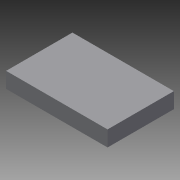
# Autodesk Inventor part: arduinoshape
Saved by Autodesk Inventor 2015 (Build 190159000, 159)
## iProperties
Created: 2015-01-29
Part Number: arduinoshape
Material: Generic
Document SubType Name: Modeling
Designer: robotics
Density: 1 g/cm^3
Appearance: Default
Author: robotics
Autodesk Inventor part; units mm, degrees
ref_plane "YZ Plane" through (0, 0, 0) normal (1, 0, 0) x (0, 1, 0)
ref_plane "XZ Plane" through (0, 0, 0) normal (0, 1, 0) x (-1, 0, 0)
ref_plane "XY Plane" through (0, 0, 0) normal (0, 0, 1) x (1, 0, 0)
sketch "Sketch2" plane through (0, 0, 0) normal (0, 1, 0) x (-1, 0, 0)
  line L0 (0, 0) -> (82.55, 0)
  line L1 (82.55, 0) -> (82.55, -53.975)
  line L2 (82.55, -53.975) -> (0, -53.975)
  line L3 (0, -53.975) -> (0, 0)
  dimension "d3" = 82.55
  dimension "d4" = 53.975
  constraints: 8 end point, 2 parallel, 1 horizontal, 1 perpendicular
  measures "d3" distance of L1.end L2.end
  measures "d4" distance of L0.end L1.end
extrude "Extrusion1" add sketch "Sketch2" along normal blind 12.7
body "Solid1"
